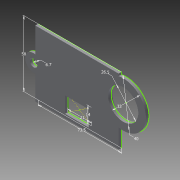
# Autodesk Inventor part: Controller_faceplate_v0.2
Saved by Autodesk Inventor 2015 (Build 190159000, 159)
## iProperties
Created: 2016-02-03
Part Number: Controller_faceplate_v0.2
Material: Generic
Document SubType Name: Modeling
Designer: wcluser
Density: 1 g/cm^3
Appearance: Default
Author: wcluser
Autodesk Inventor part; units mm, degrees
ref_plane "YZ Plane" through (0, 0, 0) normal (1, 0, 0) x (0, 1, 0)
ref_plane "XZ Plane" through (0, 0, 0) normal (0, 1, 0) x (-1, 0, 0)
ref_plane "XY Plane" through (0, 0, 0) normal (0, 0, 1) x (1, 0, 0)
sketch "Sketch1" plane through (0, 0, 0) normal (0, 1, 0) x (-1, 0, 0)
  line L0 (36.75, 29) -> (36.75, 7.0445)
  line L1 (36.75, -29) -> (-36.75, -29)
  line L2 (-36.75, -29) -> (-36.75, -12.0866)
  line L3 (-36.75, 29) -> (36.75, 29)
  line L4 (36.75, 29) -> (-36.75, -29) construction
  line L5 (36.75, -29) -> (-36.75, 29) construction
  line L6 (-36.75, 27.0891) -> (-36.75, 29)
  arc A0 (36.75, -7.6968) -> (36.75, 7.0445) centre (38.1371, -0.3261) ccw
  circle A1 centre (38.1371, -0.3261) radius 3.35
  line L7 (36.75, -7.6968) -> (36.75, -29)
  arc A2 (-36.75, 27.0891) -> (-36.75, -12.0866) centre (-40.7891, 7.5013) ccw
  circle A3 centre (-40.7891, 7.5013) radius 13.25
  arc A4 (36.75, 7.0445) -> (36.75, -7.6968) centre (38.1371, -0.3261) ccw
  arc A5 (-36.75, -12.0866) -> (-36.75, 27.0891) centre (-40.7891, 7.5013) ccw
  line L8 (10.518, -11.3105) -> (-10.482, -11.3105)
  line L9 (-10.482, -11.3105) -> (-10.482, -25.3105)
  line L10 (-10.482, -25.3105) -> (10.518, -25.3105)
  line L11 (10.518, -25.3105) -> (10.518, -11.3105)
  circle A6 centre (-40.7891, 7.5013) radius 16.5
  line L12 (-12.3133, -10.097) -> (12.3492, -10.097)
  line L13 (12.3492, -10.097) -> (12.3492, -26.5239)
  line L14 (12.3492, -26.5239) -> (-12.3133, -26.5239)
  line L15 (-12.3133, -26.5239) -> (-12.3133, -10.097)
  line L16 (-12.3133, -10.097) -> (12.3492, -26.5239) construction
  line L17 (12.3492, -10.097) -> (-12.3133, -26.5239) construction
  circle A7 centre (38.1371, -0.3261) radius 5.5
  point P0 (0, 0)
  point P1 (0.018, -18.3105)
  dimension "d0" = 58
  dimension "d1" = 73.5
  dimension "d7" = 6.7
  dimension "d8" = 40
  dimension "d9" = 26.5
  dimension "d12" = 21
  dimension "d13" = 14
  dimension "d14" = 33
  constraints: 36 end point, 9 parallel, 8 centre point, 8 point on circle, 4 coincident, 4 midpoint, 4 perpendicular, 2 concentric, 2 horizontal
  measures "d0" distance of L1.end L3.start
  measures "d1" distance of L1.start L1.end
  measures "d7" diameter of A1
  measures "d8" diameter of A2
  measures "d9" diameter of A3
  measures "d12" distance of L10.end L9.end
  measures "d13" distance of L9.end L8.end
  measures "d14" diameter of A6
extrude "Extrusion2" add sketch "Sketch1" against normal blind 2.5 contours L0 A4 L7 L1 L2 A5 L6 L3 | A0 A4 | A5 A2 | A6 | L12 L13 L14 L15 | A7
extrude "Extrusion3" add sketch "Sketch1" along normal blind 1 contours A6 | L12 L13 L14 L15 | A7
body "Solid3"
